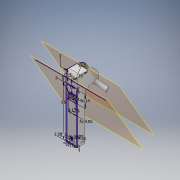
# Autodesk Inventor part: QC25BTFication_3
Saved by Autodesk Inventor 2018 (Build 220112000, 112)
## iProperties
Created: 2021-09-19
Part Number: QC25BTFication_3
Material: Generic
Document SubType Name: Modeling
Designer: dangl
Density: 1 g/cm^3
Appearance: Default
Author: dangl
Autodesk Inventor part; units mm, degrees
ref_plane "YZ Plane" through (0, 0, 0) normal (1, 0, 0) x (0, 1, 0)
ref_plane "XZ Plane" through (0, 0, 0) normal (0, 1, 0) x (-1, 0, 0)
ref_plane "XY Plane" through (0, 0, 0) normal (0, 0, 1) x (1, 0, 0)
sketch "Sketch3" plane through (0, 0, 0) normal (0, 1, 0) x (-1, 0, 0)
  line L0 (0, 0) -> (11, 0)
  line L1 (11, 0) -> (11, -56)
  line L2 (11, -56) -> (0, -56)
  line L3 (0, -56) -> (0, 0)
  line L4 (12, 1) -> (-1, 1)
  line L5 (-1, 1) -> (-1, -57)
  line L6 (-1, -57) -> (12, -57)
  line L7 (12, -57) -> (12, 1)
  line L8 (7.55, -6.2) -> (3.45, -6.2)
  line L9 (1.45, -8.2) -> (1.45, -12)
  line L10 (3.45, -14) -> (7.55, -14)
  line L11 (9.55, -12) -> (9.55, -8.2)
  arc A0 (9.55, -8.2) -> (7.55, -6.2) centre (7.55, -8.2) ccw
  arc A1 (7.55, -14) -> (9.55, -12) centre (7.55, -12) ccw
  arc A2 (1.45, -12) -> (3.45, -14) centre (3.45, -12) ccw
  arc A3 (3.45, -6.2) -> (1.45, -8.2) centre (3.45, -8.2) ccw
  circle A4 centre (5.5, -51) radius 1
  point P0 (1.45, -14)
  point P1 (1.45, -6.2)
  point P2 (9.55, -14)
  dimension "d2" = 11
  dimension "d3" = 56
  dimension "d4" = 1
  dimension "d5" = 1
  dimension "d6" = 1
  dimension "d7" = 1
  dimension "d8" = 8.1
  dimension "d9" = 7.8
  dimension "d10" = 14
  dimension "d11" = 9.55
  dimension "d12" = 2
  dimension "d30" = 2
  dimension "d31" = 5
  dimension "d32" = 5.5
  constraints: 24 end point, 8 point on circle, 8 tangent, 6 parallel, 6 point on line, 5 centre point, 3 equal radius, 3 horizontal, 3 perpendicular
  measures "d2" distance of L1.end L2.end
  measures "d3" distance of L0.end L1.end
  measures "d4" distance between parallel lines of L1 L7
  measures "d5" distance between parallel lines of L2 L6
  measures "d6" distance between parallel lines of L0 L4
  measures "d7" distance between parallel lines of L5 L3
  measures "d8" distance of point (1.45, -14) point (9.55, -14)
  measures "d9" distance of point (1.45, -6.2) point (1.45, -14)
  measures "d10" distance between parallel lines of L0 L10
  measures "d11" distance between parallel lines of L3 L11
  measures "d12" radius of A0
  measures "d30" diameter of A4
  measures "d31" distance from line of L2 A4.centre
  measures "d32" distance from line of L3 A4.centre
extrude "Extrusion1" add sketch "Sketch3" along normal blind 1.4 contours L0 L1 L2 L3
extrude "Extrusion3" add sketch "Sketch3" along normal blind 8.6 contours L7 L6 L5 L4
sketch "Sketch4" plane through (-12, 0, 1) normal (0, 0, 1) x (1, 0, 0)
  circle A0 centre (6.5, 5.4) radius 2.65
  line L0 (0, 0) -> (0, 8.6) projected
  line L1 (0, 0) -> (13, 0) projected
  point P0 (12, 0)
  dimension "d19" = 6.5
  dimension "d20" = 5.3
  dimension "d21" = 5.4
  constraints: 1 centre point
  measures "d19" distance from line of L0 A0.centre
  measures "d20" diameter of A0
  measures "d21" distance from line of L1 A0.centre
extrude "Extrusion4" cut sketch "Sketch4" against normal blind 8.6
sketch "Sketch5" plane through (1, 0, -57) normal (0, 0, -1) x (-1, 0, 0)
  line L0 (2.675, 6.25) -> (10.325, 6.25)
  line L1 (10.325, 6.25) -> (10.325, 3.55)
  line L2 (10.325, 3.55) -> (2.675, 3.55)
  line L3 (2.675, 3.55) -> (2.675, 6.25)
  line L4 (0, 0) -> (13, 0) projected
  line L5 (13, 0) -> (13, 8.6) projected
  point P0 (1, 0)
  dimension "d24" = 7.65
  dimension "d25" = 2.7
  dimension "d26" = 3.55
  dimension "d27" = 2.675
  constraints: 8 end point, 2 parallel, 1 horizontal, 1 perpendicular
  measures "d24" distance of L0.start L0.end
  measures "d25" distance of L0.end L1.end
  measures "d26" distance between parallel lines of L4 L2
  measures "d27" distance between parallel lines of L5 L1
extrude "Extrusion5" cut sketch "Sketch5" against normal blind 8.6
sketch "Sketch6" plane through (0, 0, 0) normal (0, 1, 0) x (-1, 0, 0)
  line L0 (46.885, 6) -> (-33.7151, 6)
  line L1 (12, 1) -> (-1, 1) projected
  point P0 (0, 0)
  dimension "d33" = 5
  constraints: 2 end point, 1 horizontal
  measures "d33" distance between parallel lines of L1 L0
ref_plane "Work Plane1" through (-46.885, 0, 6) normal (0, -0.8660254, -0.5) x (1, 0, 0)
ref_plane "Work Plane2" through (-46.885, 12.9904, 13.5) normal (0, -0.8660254, -0.5) x (1, 0, 0)
sketch "Sketch8" plane through (-46.885, 12.9904, 13.5) normal (0, -0.8660254, -0.5) x (1, 0, 0)
  line L0 (41.385, -17.0022) -> (58.2995, -23.1585)
  line L1 (47.885, -8.6301) -> (47.885, -58.8596) projected
  line L2 (34.885, -4.3301) -> (47.885, -4.3301) projected
  line L3 (46.885, -57.9936) -> (46.885, -9.4962) projected
  line L4 (58.2995, -23.1585) -> (59.3939, -20.1515)
  line L5 (59.3939, -20.1515) -> (42.4795, -13.9951)
  line L6 (42.4795, -13.9951) -> (41.385, -17.0022)
  point P0 (46.885, -5.1962)
  dimension "d42" = 70
  dimension "d44" = 5.5
  dimension "d45" = 18
  dimension "d46" = 3.2
  constraints: 8 end point, 2 perpendicular, 1 parallel
  measures "d42" angle of L0 L1
  measures "d44" distance from line of L3 L0.start
  measures "d45" distance of L0.start L0.end
  measures "d46" distance of L0.end L4.end
revolve "Revolution1" add sketch "Sketch8" angle 360 about axis through (-5.5, 21.4915, -1.2243) along (0.9396926, 0.1710101, -0.2961981)
sketch "Sketch11" plane through (0, 0, 0) normal (1, 0, 0) x (0, 1, 0)
  line L0 (17.1847, -15.4539) -> (-9.2723, -15.4539)
  line L1 (-9.2723, -15.4539) -> (-9.2723, -62.4336)
  line L2 (-9.2723, -62.4336) -> (17.1847, -62.4336)
  line L3 (17.1847, -62.4336) -> (17.1847, -15.4539)
  point P0 (0, 0)
  constraints: 8 end point, 2 parallel, 1 horizontal, 1 perpendicular
extrude "Extrusion8" [suppressed]
sketch "Sketch12" plane through (1, 0, 1) normal (1, 0, 0) x (0, 0, -1)
  line L0 (1.6253, 24.6) -> (3.5, 13.1)
  line L1 (3.5, 13.1) -> (5.5, 13.1)
  line L2 (5.5, 13.1) -> (6.2538, 9.6821)
  line L3 (6.2538, 9.6821) -> (12.1554, 8.6)
  line L4 (1, 8.6) -> (16.4539, 8.6)
  line L5 (0, 8.6) -> (12.1554, 8.6)
  line L6 (0, 8.6) -> (16.4539, 8.6)
  line L7 (1.6253, 24.6) -> (0, 24.6)
  line L8 (0, 24.6) -> (0, 8.6)
  point P0 (1, 0)
  dimension "d54" = 2
  dimension "d55" = 3.5
  dimension "d56" = 4.5
  dimension "d57" = 6
  dimension "d59" = 16
  constraints: 18 end point, 1 point on line
  measures "d54" distance of L0.end L1.end
  measures "d55" distance of L1.end L2.end
  measures "d56" distance between parallel lines of L4 L1
  measures "d57" distance of L2.end L3.end
  measures "d59" distance between parallel lines of L4 L7
extrude "Extrusion9" add sketch "Sketch12" against normal blind 1
sketch "Sketch13" plane through (-12, 0, 1) normal (-1, 0, 0) x (0, 0, 1)
  line L0 (0, 8.6) -> (0, 24.6)
  line L1 (0, 8.6) -> (-12.1554, 8.6) projected
  line L2 (0, 8.6) -> (-16, 8.6)
  line L3 (-58, 8.6) -> (0, 8.6) projected
  line L4 (-16, 8.6) -> (0, 24.6)
  line L5 (0, 0) -> (-58, 0) projected
  line L6 (0, 0) -> (9.5, 0)
  line L7 (12.5, 3) -> (12.5, 12.1)
  line L8 (0, 24.6) -> (0, 24.6)
  line L9 (0, 8.6) -> (0, 3)
  line L10 (-1, 1.4) -> (-1, 8.6) projected
  arc A0 (9.5, 0) -> (12.5, 3) centre (9.5, 3) ccw
  arc A1 (12.5, 12.1) -> (0, 24.6) centre (0, 12.1) ccw
  line L11 (0, 0) -> (0, 8.6) projected
  line L12 (0, 3) -> (9.5, 3)
  line L13 (9.5, 3) -> (9.5, 12.1)
  line L14 (0, 3) -> (0, 0)
  line L15 (9.5, 12.1) -> (12.5, 12.1)
  point P0 (-1, 0)
  point P1 (-16.4539, 8.6)
  point P2 (-16.4539, 0)
  point P3 (12.5, 0)
  dimension "d66" = 16
  dimension "d67" = 16
  dimension "d77" = 12.5
  dimension "d78" = 3
  dimension "d79" = 12.5
  constraints: 22 end point, 4 point on circle, 4 point on line, 4 tangent, 3 horizontal, 3 perpendicular, 2 centre point, 2 parallel, 1 vertical
  measures "d66" distance of L0.start L0.end
  measures "d67" distance of L0.start L2.end
  measures "d77" distance of L5.start point (12.5, 0)
  measures "d78" radius of A0
  measures "d79" radius of A1
extrude "Extrusion11" add sketch "Sketch13" against normal blind 1 contours L1 L2 L4 L0
sketch "Sketch14" plane through (11.4145, 24.5696, -6.5559) normal (0.9396926, 0.1710101, -0.2961981) x (-0.3006266, 0, -0.9537419)
  circle A0 centre (0, 0) radius 1.675
  line L0 (-1.675, 0) -> (-3.2, 0)
  line L1 (1.675, 0) -> (3.2, 0)
  line L2 (-3.2, 0) -> (-3.2, 3.35)
  arc A1 (-2.3221, 2.2017) -> (-1.4334, -2.861) centre (0, 0) ccw projected
  line L3 (-3.2, 3.35) -> (3.2, 3.35)
  line L4 (3.2, 3.35) -> (3.2, 0)
  point P0 (-2.8211, -22.009)
  dimension "d70" = 3.35
  dimension "d88" = 3.35
  constraints: 10 end point, 2 perpendicular, 2 point on circle, 1 centre point, 1 coincident, 1 horizontal, 1 point on line, 1 tangent, 1 vertical
  measures "d70" diameter of A0
  measures "d88" distance of L0.end L2.end
extrude "Extrusion12" cut sketch "Sketch14" against normal blind 18
sketch "Sketch15" plane through (-5.5, 21.4915, -1.2243) normal (-0.9396926, -0.1710101, 0.2961981) x (0.3006266, 0, 0.9537419)
  arc A0 (-3.2, 0) -> (3.2, 0) centre (0, 0) ccw projected
  line L0 (-1.675, 0) -> (-3.2, 0) projected
  line L1 (3.2, 0) -> (1.675, 0) projected
  arc A1 (-1.675, 0) -> (1.675, 0) centre (0, 0) ccw projected
  point P0 (2.8211, -22.009)
extrude "Extrusion13" add sketch "Sketch15" along normal up to surface surface through (-11, 0, -56) normal (-1, 0, 0)
sketch "Sketch16" plane through (-12, 0, 1) normal (0, 0, 1) x (1, 0, 0)
  line L0 (1, 17.252) -> (1, 8.6) projected
  line L1 (1, 8.6) -> (1, 5.4)
  line L2 (1, 5.4) -> (3.85, 5.4)
  circle A0 centre (6.5, 5.4) radius 2.65 projected
  line L3 (1, 8.6) -> (12, 8.6) projected
  line L4 (1, 8.6) -> (12, 8.6)
  line L5 (12, 8.6) -> (12, 5.4)
  line L6 (12, 8.6) -> (12, 1.4) projected
  line L7 (3.85, 5.4) -> (12, 5.4)
  point P0 (12, 0)
  constraints: 10 end point, 2 perpendicular, 2 point on line, 1 collinear, 1 horizontal alignment, 1 vertical, 1 other
extrude "Extrusion14" cut sketch "Sketch16" against normal blind 1.25 contours L3 L5 L7 A0 L2 L1 | A0 L7 picked at (7.2367, 6.6077)
extrude "Extrusion16" add sketch "Sketch13" against normal blind 1.5 contours L0 A1 L15 L13 L12 L9 | L12 L13 L15 L7 A0 L6 L11
sketch "Sketch17" plane through (1, 0, 1) normal (1, 0, 0) x (0, 0, -1)
  line L0 (0, 8.6) -> (0, 24.6) projected
  line L1 (0, 0) -> (0, 8.6) projected
  line L2 (58, 0) -> (-9.5, 0) projected
  arc A0 (-12.5, 3) -> (-9.5, 0) centre (-9.5, 3) ccw projected
  line L3 (-12.5, 3) -> (-12.5, 12.1) projected
  arc A1 (0, 24.6) -> (-12.5, 12.1) centre (0, 12.1) ccw projected
  point P0 (1, 0)
  point P1 (16.4539, 0)
extrude "Extrusion17" add sketch "Sketch17" against normal blind 1.5
extrude "Extrusion18" add sketch "Sketch13" against normal up to surface (11.5 mm away) contours L12 L13 L15 L7 A0 L6 L11
sketch "Sketch18" plane through (-11, 5.4, 0) normal (0, 1, 0) x (1, 0, 0)
  circle A0 centre (5.5, 1.25) radius 1.675
  line L0 (0, 15) -> (0, -1) projected
  line L1 (8.15, 0) -> (11, 0) projected
  dimension "d89" = 3.35
  dimension "d90" = 5.5
  dimension "d91" = 1.25
  constraints: 1 centre point
  measures "d89" diameter of A0
  measures "d90" distance from line of L0 A0.centre
  measures "d91" distance from line of L1 A0.centre
extrude "Extrusion19" cut sketch "Sketch18" along normal up to next
equation "\"d11\" = 0.5 * d2 + 0.5 * d8"
equation "\"d32\" = 0.5 * d2"
equation "\"d19\" = 0.5 * d2 + d4"
equation "\"d44\" = 0.5 * d2"
equation "\"d60\" = d7"
equation "\"d68\" = d4"
equation "\"d88\" = d70"
equation "\"d90\" = 0.5 * d2"
body "Solid1"
